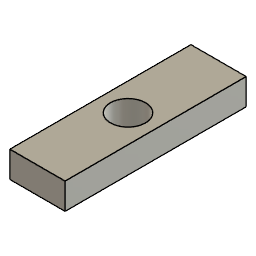
gearbox_inside_mount (Autodesk Fusion 360 design; units mm, degrees)
Autodesk Fusion 360 part; units mm, degrees
sketch "Sketch1" plane through (0, 0, 0) normal (0, 1, 0) x (1, 0, 0)
  line L0 (0, 0) -> (6, 0)
  line L1 (6, 0) -> (6, 19.6)
  line L2 (6, 19.6) -> (0, 19.6)
  line L3 (0, 19.6) -> (0, 0)
  dimension "d1" = 6
  dimension "d2" = 19.6
  constraint horizontal L0
  constraint vertical L1
  constraint horizontal L2
  constraint vertical L3
  constraint coincident L0.start L3.end
  measures "d1" distance of L0.start L0.end
  measures "d2" distance of L0.start L2.end
extrude "Extrude1" add sketch "Sketch1" along normal blind 3
sketch "Sketch2" plane through (0, 3, 0) normal (0, 1, 0) x (-1, 0, 0)
  line L0 (0, -19.6) -> (0, 0)
  line L1 (0, 0) -> (-6, 0)
  line L2 (-6, 0) -> (-6, -19.6)
  line L3 (-6, -19.6) -> (0, -19.6)
  circle A0 centre (-3, -9.8) radius 1.95
  dimension "d5" = 3.9
  measures "d5" diameter of A0
hole "Hole1" at (3, 3, -9.8) direction (0, -1, 0) diameter 4 depth 3 tip angle 180
move_face "OffsetFaces1" offset 0.1 1 faces at (3.0997, 2, -7.8025)
move_face "OffsetFaces2" offset 0.025 2 faces at (4, 2, 0) (2, 2, -19.6)
move_face "OffsetFaces3" offset -0.1 1 faces at (3, 3, -2.6167)
move_face "OffsetFaces4" offset -0.05 1 faces at (3, 2.9, -2.6167)
equation "d10 = ( 0.05 / 2 ) * 1 mm"
